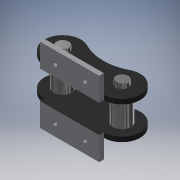
# Autodesk Inventor part: ConnectingLinks
Saved by Autodesk Inventor 2018 (Build 220112000, 112)
## iProperties
Created: 2013-07-15
Part Number: ConnectingLinks
Material: Generic
Document SubType Name: Modeling
Designer: Mill
Density: 1 g/cm^3
Appearance: Default
Author: Mill
Autodesk Inventor part; units mm, degrees
ref_plane "YZ Plane" through (0, 0, 0) normal (1, 0, 0) x (0, 1, 0)
ref_plane "XZ Plane" through (0, 0, 0) normal (0, 1, 0) x (-1, 0, 0)
sketch "Sketch1" plane through (0, 0, 0) normal (0, 0, 1) x (1, 0, 0)
  circle A0 centre (-6.35, 0) radius 3.885
  circle A1 centre (6.35, 0) radius 3.885
  arc A2 (-4.5733, 3.4549) -> (4.5733, 3.4549) centre (0, 12.3479) ccw
  line L0 (-6.35, -3.885) -> (6.35, -3.885)
  point P0 (0, 0)
  dimension "d0" = 7.77
  dimension "d1" = 6.35
  dimension "d2" = 7.77
  dimension "d3" = 6.35
  dimension "d4" = 20
  dimension "d5" = 0
  dimension "d6" = 0
  constraints: 6 point on circle, 3 centre point, 3 tangent, 2 end point, 1 horizontal
  measures "d0" diameter of A0
  measures "d1" distance of A0.centre point (0, 0)
  measures "d2" diameter of A1
  measures "d3" distance of A1.centre point (0, 0)
  measures "d4" diameter of A2
  measures "d5" vertical distance of point (0, 0) A0.centre
  measures "d6" vertical distance of point (0, 0) A1.centre
extrude "Extrusion1" add sketch "Sketch1" along normal blind 1
sketch "Sketch2" plane through (0, 0, 0) normal (0, 0, -1) x (-1, 0, 0)
  arc A0 (-4.5733, 3.4549) -> (-6.35, -3.885) centre (-6.35, 0) ccw projected
  arc A1 (6.35, -3.885) -> (4.5733, 3.4549) centre (6.35, 0) ccw projected
  circle A2 centre (-6.35, 0) radius 1.9
  circle A3 centre (6.35, 0) radius 1.9
  point P0 (-4.5733, -3.4549)
  point P1 (4.5733, -3.4549)
  point P2 (0, 0)
  dimension "d10" = 3.8
  dimension "d11" = 3.8
  constraints: 2 centre point, 2 coincident
  measures "d10" diameter of A2
  measures "d11" diameter of A3
extrude "Extrusion2" add sketch "Sketch2" along normal blind 6
sketch "Sketch3" plane through (-6.35, 0, -6) normal (0, 0, -1) x (-1, 0, 0)
  circle A0 centre (-12.7, 0) radius 1.9 projected
  circle A1 centre (0, 0) radius 1.9 projected
  arc A2 (-10.9233, 3.4549) -> (-1.7767, 3.4549) centre (-6.35, 12.3479) ccw projected
  arc A3 (-10.9233, 3.4549) -> (-12.7, -3.885) centre (-12.7, 0) ccw projected
  arc A4 (0, -3.885) -> (-1.7767, 3.4549) centre (0, 0) ccw projected
  line L0 (0, -3.885) -> (-12.7, -3.885) projected
  point P0 (-6.35, 0)
extrude "Extrusion3" add sketch "Sketch3" along normal blind 1 contours A0 | A1 | A2 A4 L0 A3
sketch "Sketch4" plane through (0, 0, 1) normal (0, 0, 1) x (1, 0, 0)
  arc A0 (-4.5733, 3.4549) -> (-6.35, -3.885) centre (-6.35, 0) ccw projected
  arc A1 (6.35, -3.885) -> (4.5733, 3.4549) centre (6.35, 0) ccw projected
  circle A2 centre (-6.35, 0) radius 1.3
  circle A3 centre (6.35, 0) radius 1.3
  point P0 (-4.5733, -3.4549)
  point P1 (4.5733, -3.4549)
  point P2 (0, 0)
  dimension "d16" = 2.6
  dimension "d17" = 2.6
  constraints: 2 centre point, 2 coincident
  measures "d16" diameter of A2
  measures "d17" diameter of A3
extrude "Extrusion4" add sketch "Sketch4" along normal blind 1
sketch "Sketch5" plane through (-6.35, 0, -7) normal (0, 0, -1) x (-1, 0, 0)
  arc A0 (-10.9233, 3.4549) -> (-12.7, -3.885) centre (-12.7, 0) ccw projected
  arc A1 (0, -3.885) -> (-1.7767, 3.4549) centre (0, 0) ccw projected
  circle A2 centre (-12.7, 0) radius 1.3
  circle A3 centre (0, 0) radius 1.3
  point P0 (-10.9233, -3.4549)
  point P1 (-1.7767, -3.4549)
  point P2 (-6.35, 0)
  dimension "d20" = 2.6
  dimension "d21" = 2.6
  constraints: 2 centre point, 2 coincident
  measures "d20" diameter of A2
  measures "d21" diameter of A3
extrude "Extrusion5" add sketch "Sketch5" along normal blind 1
chamfer "Chamfer1" distance 0.1 angle 45 2 edges at (7.65, 0, -8) (-5.05, 0, -8)
chamfer "Chamfer2" distance 0.1 angle 45 2 edges at (5.05, 0, 2) (-7.65, 0, 2)
ref_plane "Work Plane1" through (0, 0, -3) normal (0, 0, 1) x (1, 0, 0)
sketch "Skizze6" plane through (-6.35, -3.885, 0) normal (0, -1, 0) x (1, 0, 0)
  line L0 (0, 0) -> (12.7, 0)
  line L1 (12.7, 0) -> (12.7, 5)
  line L2 (12.7, 5) -> (0, 5)
  line L3 (0, 5) -> (0, 0)
  line L4 (0, -6) -> (0, -7) projected
  line L5 (0, -6) -> (12.7, -6)
  line L6 (12.7, -6) -> (12.7, -11)
  line L7 (12.7, -11) -> (0, -11)
  line L8 (0, -11) -> (0, -6)
  point P0 (6.35, 0)
  dimension "d31" = 5
  dimension "d32" = 12.7
  dimension "d33" = 12.7
  dimension "d34" = 5
  constraints: 16 end point, 4 parallel, 2 horizontal, 2 perpendicular
  measures "d31" distance of L0.end L1.end
  measures "d32" distance of L1.end L2.end
  measures "d33" distance of L6.end L7.end
  measures "d34" distance of L5.end L6.end
extrude "Extrusion6" add sketch "Skizze6" along normal blind 1
sketch "Skizze7" plane through (-6.35, -4.885, 0) normal (0, -1, 0) x (1, 0, 0)
  line L0 (6.35, 0) -> (6.35, 2.5)
  line L1 (6.35, 2.5) -> (3.175, 2.5)
  line L2 (6.35, 2.5) -> (9.525, 2.5)
  line L3 (10.9233, -6) -> (1.7767, -6) projected
  line L4 (6.35, -6) -> (6.35, -8.5)
  line L5 (6.35, -8.5) -> (3.175, -8.5)
  line L6 (6.35, -8.5) -> (9.525, -8.5)
  dimension "d37" = 2.5
  dimension "d38" = 3.175
  dimension "d39" = 3.175
  dimension "d40" = 2.5
  dimension "d41" = 3.175
  dimension "d42" = 3.175
  constraints: 12 end point, 2 horizontal, 2 perpendicular, 1 midpoint, 1 point on line, 1 vertical
  measures "d37" distance of L0.start L0.end
  measures "d38" distance of L0.end L1.end
  measures "d39" distance of L0.end L2.end
  measures "d40" distance of L4.start L4.end
  measures "d41" distance of L4.end L5.end
  measures "d42" distance of L4.end L6.end
hole "Bohrung1" at (3.175, -4.885, -8.5) at (-3.175, -4.885, -8.5) at (3.175, -4.885, 2.5) at (-3.175, -4.885, 2.5) direction (0, 1, 0) diameter 1 end through all
equation "\"d2\" = d0"
equation "\"d3\" = d1"
equation "\"d11\" = d10"
equation "\"d17\" = d16"
equation "\"d20\" = d16"
equation "\"d21\" = d16"
body "Solid1"
